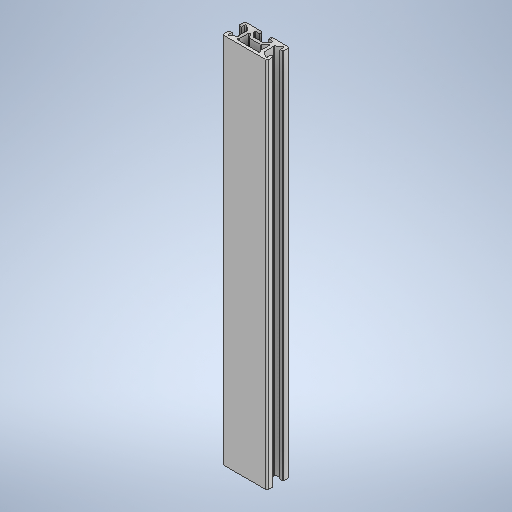
# Autodesk Inventor part: Peça2
Saved by Autodesk Inventor 2025.2 (Build 292293000, 293)
## iProperties
Created: 2025-04-03
Part Number: Peça2
Material: Genérico
Document SubType Name: Sheet Metal
Designer: kenay
Density: 1 g/cm^3
Sheet Metal Rule: Padrão_mm
Appearance: Padrão
Author: kenay
Autodesk Inventor part; units mm, degrees
ref_plane "YZ Plane" through (0, 0, 0) normal (1, 0, 0) x (0, 1, 0)
ref_plane "XZ Plane" through (0, 0, 0) normal (0, 1, 0) x (-1, 0, 0)
ref_plane "XY Plane" through (0, 0, 0) normal (0, 0, 1) x (1, 0, 0)
sketch "Esboço1" plane through (0, 0, 0) normal (0, 1, 0) x (-1, 0, 0)
  line L0 (-15, 7.5) -> (15, 7.5) construction
  line L1 (15, 7.5) -> (15, -7.5) construction
  line L2 (15, -7.5) -> (-15, -7.5) construction
  line L3 (-15, -7.5) -> (-15, 7.5) construction
  line L4 (15, 7.5) -> (-15, -7.5) construction
  line L5 (0, 7.5) -> (14, 7.5)
  arc A0 (15, 6.5) -> (14, 7.5) centre (14, 6.5) ccw
  line L6 (15, 6.5) -> (15, 3.6)
  line L7 (15, 3.6) -> (14.5, 3.6)
  line L8 (14.5, 3.6) -> (14.5, 3.1)
  line L9 (14.5, 3.1) -> (13, 3.1)
  line L10 (13, 3.1) -> (13, 5.6)
  line L11 (12.1786, 5.983) -> (9.1786, 3.4657)
  arc A1 (13, 5.6) -> (12.1786, 5.983) centre (12.5, 5.6) ccw
  arc A2 (9.1786, 3.4657) -> (9, 3.0827) centre (9.5, 3.0827) ccw
  line L12 (14, -7.5) -> (3.6, -7.5)
  line L13 (15, -3.6) -> (15, -6.5)
  arc A3 (14, -7.5) -> (15, -6.5) centre (14, -6.5) ccw
  line L14 (15, -3.6) -> (14.5, -3.6)
  line L15 (14.5, -3.6) -> (14.5, -3.1)
  line L16 (14.5, -3.1) -> (13, -3.1)
  line L17 (13, -3.1) -> (13, -5.6)
  line L18 (12.1786, -5.983) -> (9.1786, -3.4657)
  arc A4 (12.1786, -5.983) -> (13, -5.6) centre (12.5, -5.6) ccw
  line L19 (9, 3.0827) -> (9, -3.0827)
  arc A5 (9, -3.0827) -> (9.1786, -3.4657) centre (9.5, -3.0827) ccw
  line L20 (0, 5.5) -> (7.1178, 5.5)
  line L21 (0, 5.5) -> (0, 7.5)
  line L22 (13, -3.1) -> (13, 3.1) construction
  line L23 (7, -2.1501) -> (7, 4.0153)
  arc A6 (7.4392, 4.617) -> (7.1178, 5.5) centre (7.1178, 5) ccw
  arc A7 (7.1786, 4.3983) -> (7, 4.0153) centre (7.5, 4.0153) ccw
  line L24 (8.4915, 5.5) -> (7.1178, 5.5) construction
  line L25 (8.4915, 5.5) -> (7.1786, 4.3983) construction
  line L26 (7.1786, 4.3983) -> (7.4392, 4.617)
  line L27 (7, 4.0153) -> (7, -3.6) construction
  line L28 (7, -3.6) -> (3.9407, 0.3082) construction
  arc A8 (6.1063, -2.4583) -> (7, -2.1501) centre (6.5, -2.1501) ccw
  line L29 (6.1063, -2.4583) -> (3.9407, 0.3082)
  line L30 (3.547, 0.5) -> (0, 0.5)
  arc A9 (3.9407, 0.3082) -> (3.547, 0.5) centre (3.547, 0) ccw
  line L31 (0, 0.5) -> (0, -1.5)
  line L32 (0, -1.5) -> (3.0827, -1.5)
  line L33 (3.6, -7.5) -> (3.6, -7)
  line L34 (3.6, -7) -> (3.1, -7)
  line L35 (3.1, -7) -> (3.1, -5.5)
  line L36 (3.1, -5.5) -> (5.6, -5.5)
  line L37 (5.983, -4.6786) -> (3.4657, -1.6786)
  arc A10 (3.4657, -1.6786) -> (3.0827, -1.5) centre (3.0827, -2) ccw
  arc A11 (5.6, -5.5) -> (5.983, -4.6786) centre (5.6, -5) ccw
  line L38 (0, 2.5907) -> (0, -7.5) construction
  point P0 (0, 0)
  point P1 (13, -4.35)
  point P2 (13, 0)
  point P3 (9.0468, 3.294)
  dimension "d14" = 30
  dimension "d15" = 15
  dimension "d22" = 2
  dimension "d23" = 0.5
  dimension "d34" = 2.5
  dimension "d35" = 1
  dimension "d37" = 0.5
  dimension "d38" = 50
  dimension "d41" = 6
  dimension "d45" = 2
  dimension "d46" = 6.2
  dimension "d47" = 2
  dimension "d50" = 0.5
  dimension "d53" = 2
  dimension "d55" = 2
  dimension "d56" = 3.1
  dimension "d59" = 6
  dimension "d60" = 50
  dimension "d62" = 2
  dimension "d64" = 1.4656
  constraints: 79 end point, 26 point on circle, 25 tangent, 12 centre point, 11 equal length, 8 equal radius, 8 horizontal, 8 vertical, 7 perpendicular, 7 point on line, 5 midpoint, 4 collinear, 3 parallel, 1 horizontal alignment
  measures "d14" distance between parallel lines of L3 L1
  measures "d15" distance between parallel lines of L0 L2
  measures "d22" distance between parallel lines of L6 L10
  measures "d23" radius of A1
  measures "d34" distance from line of L10.end L9
  measures "d35" radius of A3
  measures "d37" distance of L14.end L15.end
  measures "d38" angle of L18 L17
  measures "d41" distance between parallel lines of L1 L19
  measures "d45" distance between parallel lines of L5 L20
  measures "d46" distance between parallel lines of L9 L16
  measures "d47" distance between parallel lines of L19 L23
  measures "d50" radius of A6
  measures "d53" distance between parallel lines of L26 L11
  measures "d55" distance of L30.end L31.end
  measures "d56" distance from line of L38.end L35
  measures "d59" distance between parallel lines of L2 L32
  measures "d60" angle of L36 L37
  measures "d62" distance between parallel lines of L2 L36
  measures "d64" distance from line of L37.start L29
extrude "Extrusão1" add sketch "Esboço1" along normal mid plane 250
mirror "Espelhar1" about plane through (0, 0, 0) normal (1, 0, 0) of "Extrusão1"
equation "\"d47\" = d45"
equation "\"Raio_vergadura\" = Espessura"
equation "\"Largura_alívio_de_vergadura\" = Espessura"
equation "\"Profundidade_alívio_de_vergadura\" = 0.5 * Espessura"
equation "\"Tamanho_alívio_de_dobra\" = 4 * Espessura"
equation "\"Remanescente_mínimo\" = 2 * Espessura"
equation "\"Raiodetransição\" = Raio_vergadura"
equation "\"Tamanho_de_raio_de_Jacobi\" = Raio_vergadura"
equation "\"TamanhoFolga\" = Espessura"
equation "\"Espessura\" = 0.5"
